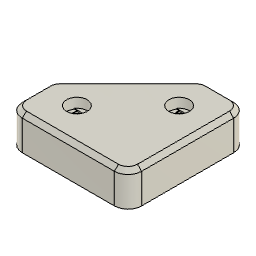
Bottom Corner Bracket - 3mm Foam Tape (Autodesk Fusion 360 design; units mm, degrees)
Autodesk Fusion 360 part; units mm, degrees
sketch "Sketch1" plane through (0, 0, 0) normal (0, 0, 1) x (1, 0, 0)
  line L0 (17.5, 17.5) -> (-17.5, 17.5)
  line L1 (-17.5, 17.5) -> (-17.5, -17.5)
  line L2 (-17.5, -17.5) -> (17.5, -17.5)
  line L3 (17.5, -17.5) -> (17.5, 17.5)
  line L4 (17.5, 17.5) -> (-17.5, -17.5) construction
  line L5 (-17.5, 17.5) -> (17.5, -17.5) construction
  line L6 (4.7, -4.7) -> (4.7, 17.5)
  line L7 (4.7, -4.7) -> (-17.5, -4.7)
  circle A0 centre (-7.5, -7.5) radius 1.7
  circle A1 centre (7.5, 7.5) radius 1.7
  line L8 (-7.5, -7.5) -> (7.5, -7.5) construction
  line L9 (7.5, -7.5) -> (7.5, 7.5) construction
  circle A2 centre (4.7, -4.7) radius 1
  dimension "d1" = 35
  dimension "d2" = 12.8
  dimension "d3" = 10
  dimension "d4" = 15
  dimension "d5" = 3.4
  dimension "d6" = 2
  constraint horizontal L0
  constraint perpendicular L0 L1
  constraint parallel L0 L2
  constraint parallel L1 L3
  constraint coincident L4 origin
  constraint coincident L5 origin
  constraint equal L1 L2
  constraint coincident L0 L6.end
  constraint perpendicular L0 L6
  constraint perpendicular L6 L7
  constraint coincident L1 L7.end
  constraint equal L6 L7
  constraint coincident A0.centre L8.start
  constraint perpendicular L3 L8
  constraint coincident L5 L8.end
  constraint perpendicular L8 L9
  constraint equal L8 L9
  constraint coincident A1.centre L9.end
  constraint equal A0 A1
  constraint coincident L6.start L7.start
  measures "d1" distance of L0.start L0.end
  measures "d2" distance of L1.end L7.end
  measures "d3" distance of L2 A0.centre
  measures "d4" distance of A0.centre L8.end
  measures "d5" diameter of A1
  measures "d6" diameter of A2
extrude "Extrude1" add sketch "Sketch1" along normal blind 6 contours L0 L1 L2 L3 L6 L7 A2
sketch "Sketch2" plane through (0, 0, 6) normal (0, 0, 1) x (-1, 0, 0)
  circle A0 centre (-7.5, -7.5) radius 1.7
  circle A1 centre (7.5, 7.5) radius 1.7
  line L0 (17.5, 4.7) -> (17.5, 17.5)
  line L1 (17.5, 17.5) -> (-17.5, 17.5)
  line L2 (-17.5, 17.5) -> (-17.5, -17.5)
  line L3 (-17.5, -17.5) -> (-4.7, -17.5)
  line L4 (-4.7, -17.5) -> (-4.7, 3.7)
  arc A2 (-3.7, 4.7) -> (-4.7, 3.7) centre (-4.7, 4.7) ccw
  line L5 (-3.7, 4.7) -> (17.5, 4.7)
  line L6 (-4.7, -17.5) -> (17.5, 4.7)
  constraint coincident L3.end L4.start
  constraint coincident L0.start L5.end
extrude "Extrude2" add sketch "Sketch2" along normal blind 4
ref_plane "WorkPlane1" through (17.5, -17.5, 5) normal (0.707107, 0.707107, 0) x (0, 0, 1)
sketch "Sketch5" plane through (17.5, -17.5, 5) normal (0.707107, 0.707107, 0) x (0, 0, 1)
  line L0 (1, -18.809) -> (1, -33.7997)
  line L1 (1, -33.7997) -> (1, -18.809)
  line L2 (1, -17.1019) -> (1, -18.809)
  line L3 (1, -33.7997) -> (2.8, -33.7997)
  line L4 (2.8, -33.7997) -> (1, -26.7997)
  dimension "d19" = 1.8
  dimension "d20" = 7
  constraint coincident L0.end L1.start
  constraint perpendicular L0 L3
  constraint coincident L0 L4.end
  measures "d19" distance of L0.end L3.end
  measures "d20" distance of L0.end L4.end
extrude "Extrude3" cut sketch "Sketch5" along normal up to surface and the other way up to surface end surface through (4.7, -3.7, 0) normal (-1, 0, 0) offset 0 second end surface through (3.7, -4.7, 0) normal (0, 1, 0) offset 0
sketch "Sketch3" plane through (0, 0, 0) normal (0, 0, -1) x (1, 0, 0)
  circle A0 centre (7.5, -7.5) radius 1.7
  circle A1 centre (-7.5, 7.5) radius 1.7
  line L0 (-17.5, 17.5) -> (-17.5, 4.7)
  line L1 (-17.5, 4.7) -> (3.7, 4.7)
  arc A2 (4.7, 3.7) -> (3.7, 4.7) centre (4.7, 4.7) ccw
  line L2 (4.7, 3.7) -> (4.7, -17.5)
  line L3 (4.7, -17.5) -> (17.5, -17.5)
  line L4 (17.5, -17.5) -> (17.5, 17.5)
  line L5 (17.5, 17.5) -> (-17.5, 17.5)
  arc A3 (17.5, 17.1) -> (17.1, 17.5) centre (17.1, 17.1) ccw
  dimension "d11" = 0.4
  constraint tangent L5 A3
  constraint coincident L5 A3.end
  constraint coincident L4 A3.start
  constraint tangent L4 A3
  measures "d11" radius of A3
sketch "Sketch4" plane through (0, 0, 10) normal (0, 0, 1) x (-1, 0, 0)
  circle A0 centre (7.5, 7.5) radius 1.7
  circle A1 centre (-7.5, -7.5) radius 1.7
  line L0 (-4.7, -17.5) -> (17.5, 4.7)
  line L1 (17.5, 4.7) -> (17.5, 17.5)
  line L2 (17.5, 17.5) -> (-17.5, 17.5)
  line L3 (-17.5, 17.5) -> (-17.5, -17.5)
  line L4 (-17.5, -17.5) -> (-4.7, -17.5)
  arc A2 (-12.1, 17.5) -> (-17.5, 12.1) centre (-12.1, 12.1) ccw
  dimension "d12" = 5.4
  constraint tangent L3 A2
  constraint coincident L3 A2.end
  constraint coincident L2 A2.start
  constraint tangent L2 A2
  measures "d12" radius of A2
fillet "Fillet2" radius 1.6 4 edges at (4.7, 17.5, 3) (4.7, -3.7, 3) (3.7, -4.7, 3) (-17.5, -4.7, 3)
fillet "Fillet1" radius 4 4 edges at (-17.5, -17.5, 5) (17.5, 17.5, 5) (-17.5, -4.7, 8.9) (4.7, 17.5, 8.9)
fillet "Fillet1" radius 4 1 edges at (17.5, -17.5, 5)
chamfer "Chamfer1" distance 1.2 angle 45 10 edges at (-6.4, 6.4, 10) (-17.1955, -4.8261, 10) (-17.5, -9.9284, 10) (-16.3284, -16.3284, 10) (0, -17.5, 10) (16.3284, -16.3284, 10) (17.5, 0, 10) (16.3284, 16.3284, 10) (9.9284, 17.5, 10) (4.8261, 17.1955, 10)
sketch "Sketch6" plane through (0, 0, 10) normal (0, 0, 1) x (-1, 0, 0)
  circle A0 centre (7.5, 7.5) radius 1.7
  circle A1 centre (-7.5, -7.5) radius 1.7
  line L0 (-16.3, 13.5) -> (-16.3, -13.5)
  arc A2 (-16.3, -13.5) -> (-13.5, -16.3) centre (-13.5, -13.5) ccw
  line L1 (-13.5, -16.3) -> (-6.3569, -16.3)
  arc A3 (-6.3569, -16.3) -> (-4.377, -15.4799) centre (-6.3569, -13.5) ccw
  line L2 (-4.377, -15.4799) -> (15.4799, 4.377)
  arc A4 (15.4799, 4.377) -> (16.3, 6.3569) centre (13.5, 6.3569) ccw
  line L3 (16.3, 6.3569) -> (16.3, 13.5)
  arc A5 (16.3, 13.5) -> (13.5, 16.3) centre (13.5, 13.5) ccw
  line L4 (13.5, 16.3) -> (-13.5, 16.3)
  circle A6 centre (7.5, 7.5) radius 3
  circle A7 centre (-7.5, -7.5) radius 3
  arc A8 (-13.5, 16.3) -> (-16.3, 13.5) centre (-13.5, 13.5) ccw
  dimension "d25" = 6
  constraint concentric A0 A6
  constraint concentric A1 A7
  constraint equal A6 A7
  measures "d25" diameter of A6
extrude "Extrude4" cut sketch "Sketch6" against normal up to surface (3 mm away) contours A6 | A7
shell "Shell1" thickness 2.6 removed faces 1 at (-2.2167, -14.6574, 0)
extrude "Extrude5" add 2 faces at (7.7827, 12.6469, 4.4) (-2.3531, -7.7827, 4.4) along direction (0, 0, -1) up to surface end surface through (0, 0, 0) normal (0, 0, -1) offset 0
sketch "Sketch7" plane through (0, 0, 7) normal (0, 0, 1) x (-1, 0, 0)
  circle A0 centre (7.5, 7.5) radius 1.7
  circle A1 centre (7.5, 7.5) radius 3
  circle A2 centre (-7.5, -7.5) radius 1.7
  circle A3 centre (-7.5, -7.5) radius 3
  line L0 (-9.9718, -5.8) -> (-5.0282, -5.8)
  line L1 (-9.9718, -9.2) -> (-5.0282, -9.2)
  line L2 (5.0282, 5.8) -> (9.9718, 5.8)
  line L3 (5.0282, 9.2) -> (9.9718, 9.2)
  constraint coincident A3 L0.start
  constraint coincident A3 L0.end
  constraint horizontal L0
  constraint coincident A3 L1.end
  constraint parallel L0 L1
  constraint coincident A1 L2.start
  constraint coincident A1 L2.end
  constraint parallel L1 L2
  constraint coincident A1 L3.start
  constraint coincident A1 L3.end
  constraint parallel L2 L3
  constraint tangent A0 L2
  constraint tangent A0 L3
  constraint tangent A2 L0
  constraint tangent A2 L1
  constraint coincident A3 L1.start
extrude "Extrude6" add sketch "Sketch7" along normal blind 0.2 contours A1 L3 | A1 L2 | A3 L0 | A3 L1
sketch "Sketch8" plane through (0, 0, 7) normal (0, 0, 1) x (-1, 0, 0)
  line L0 (-7.5, -5.8) -> (-9.9718, -5.8)
  arc A0 (-9.9718, -5.8) -> (-9.9718, -9.2) centre (-7.5, -7.5) ccw
  line L1 (-9.9718, -9.2) -> (-7.5, -9.2)
  arc A1 (-7.5, -5.8) -> (-7.5, -9.2) centre (-7.5, -7.5) ccw
  line L2 (-5.0282, -5.8) -> (-7.5, -5.8)
  arc A2 (-7.5, -9.2) -> (-7.5, -5.8) centre (-7.5, -7.5) ccw
  line L3 (-7.5, -9.2) -> (-5.0282, -9.2)
  arc A3 (-5.0282, -9.2) -> (-5.0282, -5.8) centre (-7.5, -7.5) ccw
  line L4 (7.5, 9.2) -> (5.0282, 9.2)
  arc A4 (5.0282, 9.2) -> (5.0282, 5.8) centre (7.5, 7.5) ccw
  line L5 (5.0282, 5.8) -> (7.5, 5.8)
  arc A5 (7.5, 9.2) -> (7.5, 5.8) centre (7.5, 7.5) ccw
  line L6 (9.9718, 9.2) -> (7.5, 9.2)
  arc A6 (7.5, 5.8) -> (7.5, 9.2) centre (7.5, 7.5) ccw
  line L7 (7.5, 5.8) -> (9.9718, 5.8)
  arc A7 (9.9718, 5.8) -> (9.9718, 9.2) centre (7.5, 7.5) ccw
  line L8 (-9.2, -5.8) -> (-9.2, -9.2)
  line L9 (-5.8, -5.8) -> (-5.8, -9.2)
  line L10 (9.2, 9.2) -> (9.2, 5.8)
  line L11 (5.8, 9.2) -> (5.8, 5.8)
  constraint coincident L0 L8.start
  constraint coincident L1 L8.end
  constraint perpendicular L1 L8
  constraint coincident L2 L9.start
  constraint coincident L3 L9.end
  constraint perpendicular L3 L9
  constraint coincident L6 L10.start
  constraint coincident L7 L10.end
  constraint perpendicular L7 L10
  constraint coincident L4 L11.start
  constraint coincident L5 L11.end
  constraint perpendicular L5 L11
  constraint tangent A5 L11
  constraint tangent A6 L10
  constraint tangent A2 L9
  constraint tangent A1 L8
extrude "Extrude7" cut sketch "Sketch8" against normal blind 0.2 contours L0 A1 L8 | L2 A2 L9 | L1 A1 L8 | A2 L3 L9 | L4 A5 L11 | L6 A6 L10 | L5 A5 L11 | A6 L7 L10
sketch "Sketch9" plane through (0, 0, 0) normal (0, 0, -1) x (1, 0, 0)
  line L0 (-13.5, 14.9) -> (13.5, 14.9)
  line L1 (14.9, 13.5) -> (14.9, -13.5)
  arc A0 (13.5, -14.9) -> (14.9, -13.5) centre (13.5, -13.5) ccw
  line L2 (13.5, -14.9) -> (7.3, -14.9)
  line L3 (7.3, -14.9) -> (7.3, -13.0964)
  arc A1 (7.3, -13.0964) -> (7.3, -1.9036) centre (7.5, -7.5) ccw
  line L4 (7.3, -1.9036) -> (7.3, 2.21)
  arc A2 (7.3, 2.21) -> (2.21, 7.3) centre (4.7, 4.7) ccw
  line L5 (2.21, 7.3) -> (-1.9036, 7.3)
  arc A3 (-1.9036, 7.3) -> (-13.0964, 7.3) centre (-7.5, 7.5) ccw
  line L6 (-13.0964, 7.3) -> (-14.9, 7.3)
  line L7 (-14.9, 7.3) -> (-14.9, 13.5)
  arc A4 (-13.5, 14.9) -> (-14.9, 13.5) centre (-13.5, 13.5) ccw
  circle A5 centre (-7.5, 7.5) radius 1.7
  circle A6 centre (7.5, -7.5) radius 1.7
  arc A7 (13.5, -17.5) -> (17.5, -13.5) centre (13.5, -13.5) ccw
  line L8 (17.5, -13.5) -> (17.5, 13.5)
  line L9 (13.5, 17.5) -> (-13.5, 17.5)
  arc A8 (-13.5, 17.5) -> (-17.5, 13.5) centre (-13.5, 13.5) ccw
  line L10 (-17.5, 13.5) -> (-17.5, 6.3569)
  arc A9 (-17.497, 6.2022) -> (-15.9, 4.7) centre (-15.9, 6.3) ccw
  line L11 (-15.9, 4.7) -> (2.6506, 4.7)
  arc A10 (2.6506, 4.7) -> (3.9118, 5.3154) centre (2.6506, 6.3) ccw
  arc A11 (5.3154, 3.9118) -> (3.9118, 5.3154) centre (4.7, 4.7) ccw
  arc A12 (5.3154, 3.9118) -> (4.7, 2.6506) centre (6.3, 2.6506) ccw
  line L12 (4.7, 2.6506) -> (4.7, -15.9)
  arc A13 (4.7, -15.9) -> (6.2022, -17.497) centre (6.3, -15.9) ccw
  line L13 (6.3569, -17.5) -> (13.5, -17.5)
  line L14 (4.7, -11.5) -> (10.1, -11.5)
  line L15 (10.1, -11.5) -> (10.1, -17.5)
  line L16 (-11.5, 4.7) -> (-11.5, 10.1)
  line L17 (-11.5, 10.1) -> (-17.5, 10.1)
  arc A14 (14.9, 13.5) -> (13.5, 14.9) centre (13.5, 13.5) ccw
  arc A15 (17.5, 13.5) -> (13.5, 17.5) centre (13.5, 13.5) ccw
  arc A16 (-17.5, 6.3569) -> (-17.497, 6.2022) centre (-13.5, 6.3569) ccw
  arc A17 (6.2022, -17.497) -> (6.3569, -17.5) centre (6.3569, -13.5) ccw
  dimension "d35" = 5.4
  dimension "d36" = 6
  constraint coincident L12 L14.start
  constraint perpendicular L12 L14
  constraint coincident L13 L15.end
  constraint perpendicular L13 L15
  constraint coincident L11 L16.start
  constraint perpendicular L5 L16
  constraint coincident L10 L17.end
  constraint perpendicular L10 L17
  constraint equal L14 L16
  constraint equal L15 L17
  measures "d35" distance of L14.start L14.end
  measures "d36" distance of L14.end L15.end
extrude "Extrude8" add sketch "Sketch9" along normal blind 1.4 contours A3 L6 L7 L17 | A3 L6 L7 L10 A9 L11 L16 L17 A16 | L2 L3 A1 L12 A13 L13 L14 L15 A17 | L2 L3 A1 L15
fillet "Fillet3" radius 1 6 edges at (-17.5, -10.1, -0.7) (-11.5, -10.1, -0.7) (4.7, 11.5, -0.7) (10.1, 11.5, -0.7) (10.1, 17.5, -0.7) (-11.5, -4.7, -0.7)
